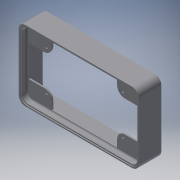
# Autodesk Inventor part: Hub Enclosure Front
Saved by Autodesk Inventor 2018 (Build 220112000, 112)
## iProperties
Created: 2018-03-22
Part Number: Hub Enclosure Front
Material: Generic
Document SubType Name: Modeling
Designer: brutu
Density: 1 g/cm^3
Appearance: Default
Author: brutu
Autodesk Inventor part; units mm, degrees
ref_plane "YZ Plane" through (0, 0, 0) normal (1, 0, 0) x (0, 1, 0)
ref_plane "XZ Plane" through (0, 0, 0) normal (0, 1, 0) x (-1, 0, 0)
ref_plane "XY Plane" through (0, 0, 0) normal (0, 0, 1) x (1, 0, 0)
sketch "Sketch1" plane through (0, 0, 0) normal (0, 0, 1) x (1, 0, 0)
  line L0 (77.5, 43.5) -> (77.5, -43.5) projected
  line L1 (77.5, -43.5) -> (-77.5, -43.5) projected
  line L2 (-77.5, -43.5) -> (-77.5, 43.5) projected
  line L3 (-77.5, 43.5) -> (77.5, 43.5) projected
  line L4 (85.48, 55.38) -> (-85.48, 55.38) projected
  arc A0 (-85.48, 55.38) -> (-96.48, 44.38) centre (-85.48, 44.38) ccw projected
  line L5 (-96.48, 44.38) -> (-96.48, -44.38) projected
  arc A1 (-96.48, -44.38) -> (-85.48, -55.38) centre (-85.48, -44.38) ccw projected
  line L6 (-85.48, -55.38) -> (85.48, -55.38) projected
  arc A2 (85.48, -55.38) -> (96.48, -44.38) centre (85.48, -44.38) ccw projected
  line L7 (96.48, -44.38) -> (96.48, 44.38) projected
  arc A3 (96.48, 44.38) -> (85.48, 55.38) centre (85.48, 44.38) ccw projected
  line L8 (-88.48, 58.38) -> (88.48, 58.38)
  line L9 (99.48, 47.38) -> (99.48, -47.38)
  line L10 (88.48, -58.38) -> (-88.48, -58.38)
  line L11 (-99.48, -47.38) -> (-99.48, 47.38)
  arc A4 (-88.48, 58.38) -> (-99.48, 47.38) centre (-88.48, 47.38) ccw
  arc A5 (99.48, 47.38) -> (88.48, 58.38) centre (88.48, 47.38) ccw
  arc A6 (88.48, -58.38) -> (99.48, -47.38) centre (88.48, -47.38) ccw
  arc A7 (-99.48, -47.38) -> (-88.48, -58.38) centre (-88.48, -47.38) ccw
  point P0 (0, 0)
  dimension "d0" = 3
  dimension "d1" = 3
  dimension "d2" = 3
  dimension "d3" = 3
  dimension "d4" = 11
  dimension "d5" = 11
  constraints: 8 end point, 8 point on circle, 8 tangent, 4 centre point, 3 equal radius, 2 parallel, 1 horizontal, 1 perpendicular
  measures "d0" distance between parallel lines of L5 L11
  measures "d1" distance between parallel lines of L4 L8
  measures "d2" distance between parallel lines of L9 L7
  measures "d3" distance between parallel lines of L10 L6
  measures "d4" radius of A4
  measures "d5" radius of A0
extrude "Extrusion1" add sketch "Sketch1" against normal blind 12 contours L0 L1 L2 L3 | A3 L7 A2 L6 A1 L5 A0 L4 | L8 A5 L9 A6 L10 A7 L11 A4
sketch "Sketch2" plane through (0, 0, 0) normal (0, 0, 1) x (1, 0, 0)
  line L0 (-88.48, 58.38) -> (88.48, 58.38) projected
  arc A0 (-88.48, 58.38) -> (-99.48, 47.38) centre (-88.48, 47.38) ccw projected
  line L1 (-99.48, -47.38) -> (-99.48, 47.38) projected
  arc A1 (-99.48, -47.38) -> (-88.48, -58.38) centre (-88.48, -47.38) ccw projected
  line L2 (88.48, -58.38) -> (-88.48, -58.38) projected
  arc A2 (88.48, -58.38) -> (99.48, -47.38) centre (88.48, -47.38) ccw projected
  line L3 (99.48, 47.38) -> (99.48, -47.38) projected
  arc A3 (99.48, 47.38) -> (88.48, 58.38) centre (88.48, 47.38) ccw projected
  line L4 (77.5, 43.5) -> (77.5, -43.5) projected
  line L5 (77.5, -43.5) -> (-77.5, -43.5) projected
  line L6 (-77.5, -43.5) -> (-77.5, 43.5) projected
  line L7 (-77.5, 43.5) -> (77.5, 43.5) projected
  line L8 (85.48, 55.38) -> (-85.48, 55.38) projected
  arc A4 (-85.48, 55.38) -> (-96.48, 44.38) centre (-85.48, 44.38) ccw projected
  line L9 (-96.48, 44.38) -> (-96.48, -44.38) projected
  arc A5 (-96.48, -44.38) -> (-85.48, -55.38) centre (-85.48, -44.38) ccw projected
  line L10 (-85.48, -55.38) -> (85.48, -55.38) projected
  arc A6 (85.48, -55.38) -> (96.48, -44.38) centre (85.48, -44.38) ccw projected
  line L11 (96.48, -44.38) -> (96.48, 44.38) projected
  arc A7 (96.48, 44.38) -> (85.48, 55.38) centre (85.48, 44.38) ccw projected
  arc A8 (-85.48, 56.38) -> (-97.48, 44.38) centre (-85.48, 44.38) ccw
  line L12 (-85.48, 56.38) -> (85.48, 56.38)
  arc A9 (97.48, 44.38) -> (85.48, 56.38) centre (85.48, 44.38) ccw
  line L13 (97.48, 44.38) -> (97.48, -44.38)
  arc A10 (85.48, -56.38) -> (97.48, -44.38) centre (85.48, -44.38) ccw
  line L14 (85.48, -56.38) -> (-85.48, -56.38)
  arc A11 (-97.48, -44.38) -> (-85.48, -56.38) centre (-85.48, -44.38) ccw
  line L15 (-97.48, -44.38) -> (-97.48, 44.38)
  point P0 (0, 0)
  dimension "d8" = 1
  constraints: 8 end point, 8 point on circle, 4 centre point, 7 other
  measures "d8" radial gap between concentric circles of A4 A8
extrude "Extrusion2" cut sketch "Sketch2" against normal blind 1.5 contours L4 L5 L6 L7 | A7 L11 A6 L10 A5 L9 A4 L8 | L12 A9 L13 A10 L14 A11 L15 A8
sketch "Sketch3" plane through (0, 0, -1.5) normal (0, 0, 1) x (1, 0, 0)
  arc A0 (-85.48, 56.38) -> (-97.48, 44.38) centre (-85.48, 44.38) ccw projected
  line L0 (-97.48, -44.38) -> (-97.48, 44.38) projected
  arc A1 (-97.48, -44.38) -> (-85.48, -56.38) centre (-85.48, -44.38) ccw projected
  line L1 (85.48, -56.38) -> (-85.48, -56.38) projected
  arc A2 (85.48, -56.38) -> (97.48, -44.38) centre (85.48, -44.38) ccw projected
  line L2 (97.48, 44.38) -> (97.48, -44.38) projected
  arc A3 (97.48, 44.38) -> (85.48, 56.38) centre (85.48, 44.38) ccw projected
  line L3 (-85.48, 56.38) -> (85.48, 56.38) projected
  arc A4 (-85.48, 54.38) -> (-95.48, 44.38) centre (-85.48, 44.38) ccw
  line L4 (-85.48, 54.38) -> (85.48, 54.38)
  arc A5 (95.48, 44.38) -> (85.48, 54.38) centre (85.48, 44.38) ccw
  line L5 (95.48, 44.38) -> (95.48, -44.38)
  arc A6 (85.48, -54.38) -> (95.48, -44.38) centre (85.48, -44.38) ccw
  line L6 (85.48, -54.38) -> (-85.48, -54.38)
  arc A7 (-95.48, -44.38) -> (-85.48, -54.38) centre (-85.48, -44.38) ccw
  line L7 (-95.48, -44.38) -> (-95.48, 44.38)
  point P0 (0, 0)
  dimension "d11" = 2
  constraints: 8 end point, 8 point on circle, 4 centre point, 7 other
  measures "d11" radial gap between concentric circles of A0 A4
extrude "Extrusion3" cut sketch "Sketch3" against normal blind 9.9 contours L4 A5 L5 A6 L6 A7 L7 A4
fillet "Fillet1" radius 3.175 8 edges at (92.5511, 51.4511, -11.4) (95.48, 0, -11.4) (92.5511, -51.4511, -11.4) (0, -54.38, -11.4) (-92.5511, -51.4511, -11.4) (-95.48, 0, -11.4) (-92.5511, 51.4511, -11.4) (0, 54.38, -11.4)
sketch "Sketch5" plane through (0, 0, -12) normal (0, 0, -1) x (-1, 0, 0)
  arc A0 (-85.48, 51.205) -> (-92.305, 44.38) centre (-85.48, 44.38) ccw projected
  line L0 (85.48, 51.205) -> (-85.48, 51.205) projected
  arc A1 (92.305, 44.38) -> (85.48, 51.205) centre (85.48, 44.38) ccw projected
  line L1 (92.305, -44.38) -> (92.305, 44.38) projected
  arc A2 (85.48, -51.205) -> (92.305, -44.38) centre (85.48, -44.38) ccw projected
  line L2 (-85.48, -51.205) -> (85.48, -51.205) projected
  arc A3 (-92.305, -44.38) -> (-85.48, -51.205) centre (-85.48, -44.38) ccw projected
  line L3 (-92.305, 44.38) -> (-92.305, -44.38) projected
  circle A4 centre (-63.1, 33.8) radius 1.5 projected
  circle A5 centre (-63.1, -31.85) radius 1.5 projected
  circle A6 centre (63.1, -31.85) radius 1.5 projected
  circle A7 centre (63.1, 33.8) radius 1.5 projected
  circle A8 centre (-63.1, 33.8) radius 1.905
  circle A9 centre (63.1, 33.8) radius 1.905
  circle A10 centre (63.1, -31.85) radius 1.905
  circle A11 centre (-63.1, -31.85) radius 1.905
  line L4 (-54.205, 51.205) -> (-54.205, 38.505)
  line L5 (-66.905, 25.805) -> (-92.305, 25.805)
  arc A12 (-66.905, 25.805) -> (-54.205, 38.505) centre (-66.905, 38.505) ccw
  line L6 (0, 51.205) -> (0, -51.205)
  line L7 (-92.305, 0) -> (92.305, 0)
  line L8 (54.205, 51.205) -> (54.205, 38.505)
  line L9 (66.905, 25.805) -> (92.305, 25.805)
  arc A13 (54.205, 38.505) -> (66.905, 25.805) centre (66.905, 38.505) ccw
  line L10 (-54.205, -51.205) -> (-54.205, -38.505)
  line L11 (-66.905, -25.805) -> (-92.305, -25.805)
  arc A14 (-54.205, -38.505) -> (-66.905, -25.805) centre (-66.905, -38.505) ccw
  line L12 (54.205, -51.205) -> (54.205, -38.505)
  arc A15 (66.905, -25.805) -> (54.205, -38.505) centre (66.905, -38.505) ccw
  line L13 (66.905, -25.805) -> (92.305, -25.805)
  line L14 (-54.205, 51.205) -> (54.205, 51.205)
  line L15 (92.305, 25.805) -> (92.305, -25.805)
  line L16 (54.205, -51.205) -> (-54.205, -51.205)
  line L17 (-92.305, -25.805) -> (-92.305, 25.805)
  point P0 (0, 0)
  dimension "d38" = 3.81
  dimension "d39" = 3.81
  dimension "d40" = 3.81
  dimension "d41" = 3.81
  dimension "d51" = 12.7
  dimension "d52" = 25.4
  dimension "d53" = 38.1
  constraints: 28 end point, 15 symmetric about line, 8 centre point, 8 point on circle, 4 coincident, 4 midpoint, 3 collinear, 2 point on line, 2 tangent, 1 horizontal, 1 perpendicular, 1 vertical, 3 other
  measures "d38" diameter of A8
  measures "d39" diameter of A9
  measures "d40" diameter of A10
  measures "d41" diameter of A11
  measures "d51" radius of A12
  measures "d52" distance between parallel lines of L0 L5
  measures "d53" distance between parallel lines of L3 L4
extrude "Extrusion4" cut sketch "Sketch5" against normal through all contours L0 L6 L7 L3 L5 A12 L4 | L0 L8 A13 L9 L1 L7 L6 | L7 L6 L2 L10 A14 L11 L3 | L7 L1 L13 A15 L12 L2 L6 | A4 | A5 | A6 | A7 | A8 | A9 | A10 | A11
equation "\"d1\" = d0"
equation "\"d2\" = d0"
equation "\"d3\" = d0"
equation "\"d4\" = d5"
equation "\"d39\" = d38"
equation "\"d40\" = d38"
equation "\"d41\" = d38"
body "Solid1"
